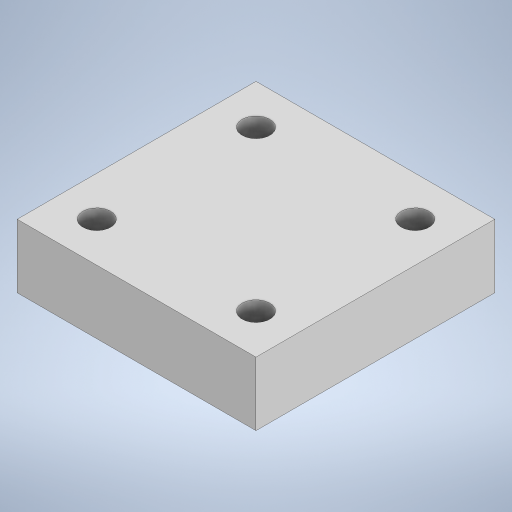
# Autodesk Inventor part: 4_center_union
Saved by Autodesk Inventor 2023 (Build 270158000, 158)
## iProperties
Created: 2022-12-26
Part Number: 4_center_union
Material: Genérico
Document SubType Name: Modeling
Designer: inigo
Density: 1 g/cm^3
Appearance: Valor por defecto
Author: inigo
Autodesk Inventor part; units mm, degrees
ref_plane "YZ Plane" through (0, 0, 0) normal (1, 0, 0) x (0, 1, 0)
ref_plane "XZ Plane" through (0, 0, 0) normal (0, 1, 0) x (-1, 0, 0)
ref_plane "XY Plane" through (0, 0, 0) normal (0, 0, 1) x (1, 0, 0)
sketch "Boceto1" plane through (0, 0, 0) normal (0, 1, 0) x (-1, 0, 0)
  line L0 (15, 15) -> (-15, 15)
  line L1 (-15, 15) -> (-15, -15)
  line L2 (-15, -15) -> (15, -15)
  line L3 (15, -15) -> (15, 15)
  line L4 (15, 15) -> (-15, -15) construction
  line L5 (-15, 15) -> (15, -15) construction
  circle A0 centre (-10, -10) radius 1.75
  line L6 (0, 0) -> (0, 4.5842)
  line L7 (0, 0) -> (-4.6861, 0)
  circle A1 centre (-10, 10) radius 1.75
  line L8 (15, 15) -> (-15, -15) construction
  circle A2 centre (10, -10) radius 1.75
  circle A3 centre (10, 10) radius 1.75
  dimension "d0" = 30
  dimension "d1" = 30
  dimension "d2" = 3.5
  dimension "d3" = 10
  dimension "d4" = 10
  constraints: 18 end point, 4 centre point, 3 symmetric about line, 2 horizontal, 2 midpoint, 2 parallel, 1 perpendicular, 1 vertical, 3 other
  measures "d0" distance of L2.end L1.end
  measures "d1" distance of L1.end L0.end
  measures "d2" diameter of A0
  measures "d3" distance from line of L6 A0.centre
  measures "d4" distance from line of A0.centre L7
extrude "Extrusión1" add sketch "Boceto1" along normal blind 8
